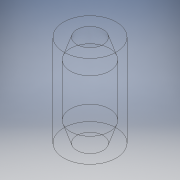
# Autodesk Inventor part: 기본 투상 연습5
Saved by Autodesk Inventor 2018.3 (Build 223284000, 284)
## iProperties
Created: 2019-10-08
Part Number: 기본 투상 연습5
Material: 일반
Document SubType Name: Modeling
Designer: MyTool
Density: 1 g/cm^3
Appearance: 기본값
Author: MyTool
Autodesk Inventor part; units mm, degrees
ref_plane "YZ Plane" through (0, 0, 0) normal (1, 0, 0) x (0, 1, 0)
ref_plane "XZ Plane" through (0, 0, 0) normal (0, 1, 0) x (-1, 0, 0)
ref_plane "XY Plane" through (0, 0, 0) normal (0, 0, 1) x (1, 0, 0)
sketch "스케치3" plane through (0, 0, 0) normal (1, 0, 0) x (0, 1, 0)
  line L0 (0, 0) -> (0, -70)
  line L1 (0, -70) -> (10, -70)
  line L2 (10, -70) -> (20, -70)
  line L3 (20, -70) -> (20, 0)
  line L4 (20, 0) -> (10, 0)
  line L5 (10, 0) -> (15, -15)
  line L6 (15, -15) -> (15, -55)
  line L7 (15, -55) -> (10, -70)
  dimension "d10" = 70
  dimension "d11" = 10
  dimension "d12" = 10
  dimension "d13" = 70
  dimension "d14" = 10
  dimension "d15" = 15
  dimension "d16" = 15
  dimension "d17" = 40
  constraints: 16 end point, 2 perpendicular, 1 horizontal, 1 parallel, 1 point on line, 1 vertical
  measures "d10" distance of L0.start L0.end
  measures "d11" distance of L0.end L1.end
  measures "d12" distance of L1.end L2.end
  measures "d13" distance of L2.end L3.end
  measures "d14" distance of L3.end L4.end
  measures "d15" distance between parallel lines of L0 L6
  measures "d16" vertical distance of L6.end L1.end
  measures "d17" distance of L5.end L6.end
revolve "회전2" add sketch "스케치3" angle 360 about axis through (0, 0, 0) along (0, 0, -1)
